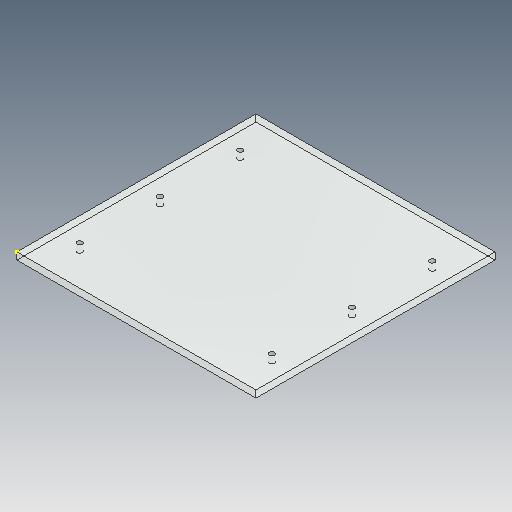
# Autodesk Inventor part: acrylic_base
Saved by Autodesk Inventor 2025.4 (Build 294407020, 407B)
## iProperties
Created: 2026-09-08
Part Number: acrylic_base
Material: Generic
Document SubType Name: Modeling
Designer: Aiden
Density: 1 g/cm^3
Appearance: Default
Author: Aiden
Autodesk Inventor part; units mm, degrees
ref_plane "YZ Plane" through (0, 0, 0) normal (1, 0, 0) x (0, 1, 0)
ref_plane "XZ Plane" through (0, 0, 0) normal (0, 1, 0) x (-1, 0, 0)
ref_plane "XY Plane" through (0, 0, 0) normal (0, 0, 1) x (1, 0, 0)
sketch "Sketch1" plane through (0, 0, 0) normal (0, 1, 0) x (-1, 0, 0)
  line L0 (0, 0) -> (-304.8, 0)
  line L1 (-304.8, 0) -> (-304.8, -304.8)
  line L2 (-304.8, -304.8) -> (0, -304.8)
  line L3 (0, -304.8) -> (0, 0)
  dimension "d0" = 304.8
  dimension "d1" = 304.8
  constraints: 8 end point, 2 parallel, 1 horizontal, 1 perpendicular
  measures "d0" distance of L1.end L2.end
  measures "d1" distance of L2.end L0.start
extrude "Extrusion1" add sketch "Sketch1" along normal blind 9
sketch "Sketch2" plane through (0, 9, 0) normal (0, 1, 0) x (1, 0, 0)
  point P0 (0, 0)
sketch "Sketch3" plane through (0, 9, 0) normal (0, 1, 0) x (1, 0, 0)
  line L0 (304.8, 304.8) -> (0, 304.8) projected
  line L1 (152.4, 304.8) -> (152.4, 0) construction
  line L2 (0, 0) -> (304.8, 0) projected
  line L3 (30, 304.8) -> (30, 0) construction
  line L4 (0, 304.8) -> (0, 0) projected
  point P0 (30, 254.8)
  point P1 (30, 152.4)
  point P2 (30, 50)
  point P3 (274.8, 254.8)
  point P4 (274.8, 152.4)
  point P5 (274.8, 50)
  dimension "d4" = 30
  dimension "d5" = 50
  dimension "d6" = 50
  constraints: 4 end point, 4 point on line, 3 midpoint, 3 symmetric about line, 1 perpendicular
  measures "d4" distance between parallel lines of L4 L3
  measures "d5" distance from line of L0 point (30, 254.8)
  measures "d6" distance from line of L2 point (30, 50)
hole "Hole1" at (30, 9, -254.8) at (274.8, 9, -254.8) at (274.8, 9, -152.4) at (30, 9, -152.4) at (30, 9, -50) at (274.8, 9, -50) direction (0, -1, 0) diameter 6.604 end through all
body "Solid1"
